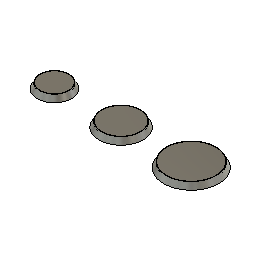
Warhammer Model Bases v6 (Autodesk Fusion 360 design; units mm, degrees)
Autodesk Fusion 360 part; units mm, degrees
note: some values were not read from the file. Chosen so that the rebuilt part matches the saved one: which bodies a step acts on.
sketch "Base" plane through (0, 0, 0) normal (0, 1, 0) x (1, 0, 0)
  circle A0 centre (0, 0) radius 12.5
  circle A1 centre (0, 0) radius 6.5
  circle A2 centre (48.26, 0) radius 16
  circle A3 centre (48.26, 0) radius 6.5
  circle A4 centre (99.06, 0) radius 20
  circle A5 centre (99.06, 0) radius 6.5
  dimension "d1" = 25
  dimension "d2" = 13
  dimension "d3" = 32
  dimension "d4" = 13
  dimension "d5" = 40
  dimension "d6" = 13
  constraint coincident A0.centre A1.centre
  constraint concentric A0 A1
  constraint concentric A2 A3
  constraint concentric A4 A5
  measures "d1" diameter of A0
  measures "d2" diameter of A1
  measures "d3" diameter of A2
  measures "d4" diameter of A3
  measures "d5" diameter of A4
  measures "d6" diameter of A5
extrude "Extrude1" add sketch "Base" along normal blind 4 contours A0 | A1 | A2 | A3 | A4 | A5 makes body 1 at (-3.3879, 0, 0.621) makes body 2 at (51.5853, 0, 4.1698) makes body 3 at (104.2042, 0, 1.1021)
chamfer "Chamfer1" distance 2 distance2 4 3 edges at (-11.6541, 4, 4.5202) (80.4135, 4, 7.2323) (33.3428, 4, 5.7858) measured on face at (-3.3879, 4, 0.621) measured on face at (104.2042, 4, 1.1021) measured on face at (51.5853, 4, 4.1698) on bodies 1 2 3
extrude "Extrude2" cut sketch "Base" along normal blind 2 contours A1 | A3 | A5 bodies 1 2 3
copy_body "CopyPasteBodies1" bodies 1 2 3 makes body 4 makes body 5 makes body 6
move_body "Move1" bodies 4 5 6 to x (1, 0, 0) y (0, 1, 0) z (0, 0, 1) at (0, 0, 58.42)
extrude "Extrude3" add 3 faces at (1.9521, 2, 0.9401) (46.5997, 2, 2.4353) (93.9784, 2, -0.1027) along direction (0, -1, 0) up to surface end surface through (0, 0, 0) normal (0, -1, 0) offset 0 on bodies 1 2 3 bodies 1 2 3
extrude "Extrude4" cut sketch "Base" along normal blind 1 and the other way blind -3 contours A1 | A3 | A5 bodies 1 2 3
sketch "Pocket Cut Profile" plane through (0, 0, 0) normal (0, 0, 1) x (1, 0, 0)
  line L0 (6.5, 1) -> (-6.5, 1)
  line L1 (6.5, 3) -> (-6.5, 3)
  line L2 (54.76, 1) -> (41.76, 1)
  line L3 (54.76, 3) -> (41.76, 3)
  line L4 (105.56, 1) -> (92.56, 1)
  line L5 (105.56, 3) -> (92.56, 3)
  line L6 (-6.5, 3) -> (-6.5, 1)
  line L7 (6.5, 3) -> (6.5, 1)
  line L8 (41.76, 3) -> (41.76, 1)
  line L9 (54.76, 3) -> (54.76, 1)
  line L10 (92.56, 3) -> (92.56, 1)
  line L11 (105.56, 3) -> (105.56, 1)
  line L12 (6.4, 1.1) -> (-6.4, 1.1)
  line L13 (-6.4, 2.9) -> (-6.4, 1.1)
  line L14 (6.4, 2.9) -> (-6.4, 2.9)
  line L15 (6.4, 2.9) -> (6.4, 1.1)
  line L16 (54.66, 2.9) -> (54.66, 1.1)
  line L17 (54.66, 1.1) -> (41.86, 1.1)
  line L18 (41.86, 2.9) -> (41.86, 1.1)
  line L19 (54.66, 2.9) -> (41.86, 2.9)
  line L20 (105.46, 2.9) -> (105.46, 1.1)
  line L21 (105.46, 1.1) -> (92.66, 1.1)
  line L22 (92.66, 2.9) -> (92.66, 1.1)
  line L23 (105.46, 2.9) -> (92.66, 2.9)
  dimension "d19" = 0.1
  dimension "d20" = 0.1
  dimension "d21" = 0.1
  constraint coincident L1.end L6.start
  constraint coincident L0.end L6.end
  constraint coincident L1.start L7.start
  constraint coincident L0.start L7.end
  constraint coincident L3.end L8.start
  constraint coincident L2.end L8.end
  constraint coincident L3.start L9.start
  constraint coincident L2.start L9.end
  constraint coincident L5.end L10.start
  constraint coincident L4.end L10.end
  constraint coincident L5.start L11.start
  constraint coincident L4.start L11.end
extrude "Extrude5" cut sketch "Pocket Cut Profile" along normal blind 29.3688 bodies 1 2 3 makes body 9 at (95.1577, 1.1, 14.5895) makes body 8 at (49.1497, 1.1, 12.409) makes body 7 at (0.7199, 1.1, 10.0881)
copy_body "CopyPasteBodies2" bodies 4 6 5 makes body 10 makes body 11 makes body 12
move_body "Move2" bodies 10 11 12 to x (1, 0, 0) y (0, 1, 0) z (0, 0, 1) at (0, 0, 78.74)
extrude "Extrude6" add 3 faces at (1.6711, 2, 135.4178) (46.5997, 2, 139.5953) (103.23, 2, 138.9237) along direction (0, -1, 0) up to surface end surface through (0, 0, 137.16) normal (0, -1, 0) offset 0 on bodies 10 11 12 bodies 10 11 12
ref_plane "WorkPlane1" through (0, -4, 137.16) normal (0, 0, 1) x (1, 0, 0)
sketch "Top Load Cut Profile" plane through (0, -4, 137.16) normal (0, 0, 1) x (1, 0, 0)
  line L0 (12.5, 4) -> (-12.5, 4)
  line L1 (-10.5, 8) -> (10.5, 8)
  line L2 (64.26, 4) -> (32.26, 4)
  line L3 (34.26, 8) -> (62.26, 8)
  line L4 (119.06, 4) -> (79.06, 4)
  line L5 (81.06, 8) -> (117.06, 8)
  line L6 (-10.5, 8) -> (-10.5, 7.1)
  line L7 (-10.5, 7.1) -> (-6, 7.1)
  line L8 (-6, 7.1) -> (-6, 5)
  line L9 (-6, 5) -> (0, 5)
  line L10 (0, 5) -> (0, 8)
  line L11 (34.26, 8) -> (34.26, 7.1)
  line L12 (34.26, 7.1) -> (42.26, 7.1)
  line L13 (42.26, 7.1) -> (42.26, 5)
  line L14 (42.26, 5) -> (48.26, 5)
  line L15 (48.26, 5) -> (48.26, 8)
  line L16 (81.06, 8) -> (81.06, 7.1)
  line L17 (81.06, 7.1) -> (93.06, 7.1)
  line L18 (93.06, 7.1) -> (93.06, 5)
  line L19 (93.06, 5) -> (99.06, 5)
  line L20 (99.06, 5) -> (99.06, 8)
  line L21 (99.06, 0) -> (99.06, 8)
  line L22 (0, 8) -> (-10.2, 8)
  line L23 (-10.2, 8) -> (-10.2, 7.2)
  line L24 (-10.2, 7.2) -> (0, 7.2)
  line L25 (0, 7.2) -> (0, 8)
  line L26 (48.26, 8) -> (34.56, 8)
  line L27 (34.56, 8) -> (34.56, 7.2)
  line L28 (34.56, 7.2) -> (48.26, 7.2)
  line L29 (48.26, 7.2) -> (48.26, 8)
  line L30 (99.06, 8) -> (81.36, 8)
  line L31 (81.36, 8) -> (81.36, 7.2)
  line L32 (81.36, 7.2) -> (99.06, 7.2)
  line L33 (99.06, 7.2) -> (99.06, 8)
  line L34 (119.06, 4) -> (79.06, 4)
  line L35 (64.26, 4) -> (32.26, 4)
  line L36 (12.5, 4) -> (-12.5, 4)
  dimension "d26" = 6
  dimension "d27" = 2.1
  dimension "d28" = 0.9
  dimension "d29" = 90
  dimension "d31" = 2.1
  dimension "d32" = 6
  dimension "d33" = 6
  dimension "d34" = 90
  dimension "d35" = 2.1
  dimension "d36" = 0.1
  dimension "d37" = 0.3
  dimension "d38" = 0.1
  dimension "d39" = 0.3
  dimension "d40" = 0.1
  dimension "d41" = 0.3
  dimension "d45" = 36
  dimension "d46" = 40
  dimension "d47" = 28
  dimension "d48" = 32
  dimension "d49" = 21
  dimension "d50" = 25
  dimension "d51" = 4
  constraint coincident L1.start L6.start
  constraint perpendicular L1 L6
  constraint perpendicular L6 L7
  constraint perpendicular L7 L8
  constraint perpendicular L6 L9
  constraint midpoint L1 L10.end
  constraint perpendicular L1 L10
  constraint coincident L3.start L11.start
  constraint perpendicular L3 L11
  constraint perpendicular L11 L12
  constraint perpendicular L12 L13
  constraint perpendicular L13 L14
  constraint midpoint L3 L15.end
  constraint perpendicular L3 L15
  constraint equal L6 L11
  constraint equal L9 L14
  constraint equal L8 L13
  constraint coincident L5.start L16.start
  constraint perpendicular L5 L16
  constraint perpendicular L16 L17
  constraint perpendicular L17 L18
  constraint perpendicular L18 L19
  constraint midpoint L5 L20.end
  constraint equal L11 L16
  constraint equal L14 L19
  constraint equal L13 L18
  constraint horizontal L22
  constraint vertical L23
  constraint horizontal L24
  constraint vertical L25
  constraint horizontal L26
  constraint vertical L27
  constraint horizontal L28
  constraint vertical L29
  constraint horizontal L30
  constraint vertical L31
  constraint horizontal L32
  constraint vertical L33
  constraint coincident L20.end L21.end
  measures "d26" distance of L8.end L9.end
  measures "d27" distance of L7 L9
  measures "d28" distance of L1 L7
  measures "d29" angle of L5 L20
  measures "d31" distance of L12.end L13.end
  measures "d32" distance of L13.end L14.end
  measures "d33" distance of L18 L21
  measures "d34" angle of L18 L19
  measures "d35" distance of L17.end L18.end
  measures "d36" distance of L7 L24
  measures "d37" distance of L6 L23
  measures "d38" distance of L12 L28
  measures "d39" distance of L11 L27
  measures "d40" distance of L17 L32
  measures "d41" distance of L16 L31
  measures "d45" distance of L5.start L5.end
  measures "d46" distance of L4.start L4.end
  measures "d47" distance of L3.start L3.end
  measures "d48" distance of L2.start L2.end
  measures "d49" distance of L1.start L1.end
  measures "d50" distance of L0.start L0.end
  measures "d51" distance of L5 L34
revolve "Revolve1" cut sketch "Top Load Cut Profile" angle 360 about axis through (48.26, 1, 137.16) along (0, 1, 0) contours L3 L11 L12 L13 L14 L15 L27 L28 bodies 12 makes body 13 at (52.9621, 0, 132.1953)
revolve "Revolve2" cut sketch "Top Load Cut Profile" angle 360 about axis through (0, 1, 137.16) along (0, 1, 0) contours L1 L6 L7 L8 L9 L10 L23 L24 bodies 10 makes body 14 at (-3.3879, 0, 137.781)
revolve "Revolve3" cut sketch "Top Load Cut Profile" angle 360 about axis through (99.06, -4, 137.16) along (0, 1, 0) contours L5 L16 L17 L18 L19 L20 L21 L31 L32 bodies 11 makes body 15 at (96.2604, 0, 135.8118)
delete_body "RemoveBody1" bodies 1
delete_body "RemoveBody2" bodies 5
delete_body "RemoveBody3" bodies 2
delete_body "RemoveBody4" bodies 3
delete_body "RemoveBody5" bodies 4
delete_body "RemoveBody6" bodies 6
delete_body "RemoveBody7" bodies 8
delete_body "RemoveBody8" bodies 7
delete_body "RemoveBody9" bodies 9
equation "d13 = 0\""
equation "d18 = 0.0 °"
equation "d22 = 1 5/32\""
equation "d24 = 0\""
equation "d29 = 90 °"
equation "d34 = 90.0 °"
named bodies: "25mm Base Pocket", "32mm Base Pocket", "40mm Base Pocket", "25mm Base", "32mm Base", "40mm Base", "25mm Base (1)", "32mm Base (1)", "40mm Base (1)", "25mm Base Plug", "32mm Base Plug", "40mm Base Plug", "25mm Top Load Cap", "40mm Top Load Cap", "32mm Top Load Cap", "32mm Base Top Load", "25mm Base Top Load", "40mm Base Top Load"
